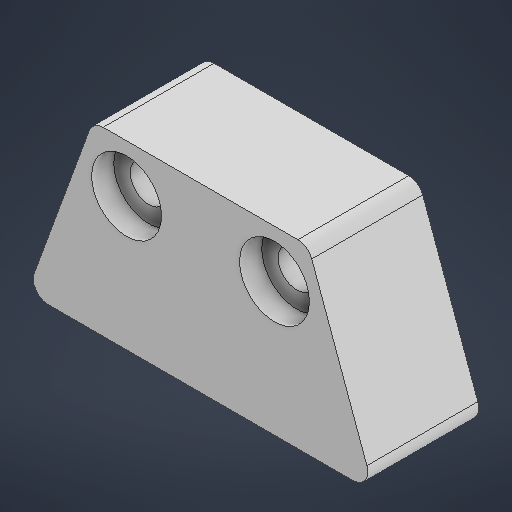
# Autodesk Inventor part: EngineMount
Saved by Autodesk Inventor 2025.3 (Build 293356030, 356C)
## iProperties
Created: 2025-10-14
Part Number: EngineMount
Material: Generic
Document SubType Name: Modeling
Designer: yo
Density: 1 g/cm^3
Appearance: Default
Author: yo
Autodesk Inventor part; units mm, degrees
ref_plane "YZ Plane" through (0, 0, 0) normal (1, 0, 0) x (0, 1, 0)
ref_plane "XZ Plane" through (0, 0, 0) normal (0, 1, 0) x (-1, 0, 0)
ref_plane "XY Plane" through (0, 0, 0) normal (0, 0, 1) x (1, 0, 0)
sketch "Sketch1" plane through (0, 0, 0) normal (0, 0, 1) x (1, 0, 0)
  line L0 (-41.2246, 0) -> (41.2246, 0)
  line L1 (-26.3201, 48.95) -> (26.3201, 48.95)
  circle A0 centre (-20, 36) radius 9.45
  line L2 (0, 48.95) -> (0, 0) construction
  circle A1 centre (-20, 36) radius 5
  circle A2 centre (20, 36) radius 9.45
  circle A3 centre (20, 36) radius 5
  arc A4 (-44.9834, 5.3681) -> (-41.2246, 0) centre (-41.2246, 4) ccw
  arc A5 (-26.3201, 48.95) -> (-30.0788, 46.3181) centre (-26.3201, 44.95) ccw
  line L3 (-44.9834, 5.3681) -> (-30.0788, 46.3181)
  arc A6 (41.2246, 0) -> (44.9834, 5.3681) centre (41.2246, 4) ccw
  arc A7 (30.0788, 46.3181) -> (26.3201, 48.95) centre (26.3201, 44.95) ccw
  line L4 (44.9834, 5.3681) -> (30.0788, 46.3181)
  dimension "d1" = 18.9
  dimension "d3" = 3.5
  dimension "d4" = 36
  dimension "d7" = 10
  dimension "d8" = 40
  dimension "d10" = 4
  dimension "d11" = 13
  dimension "d12" = 70
  constraints: 10 end point, 8 centre point, 8 point on circle, 6 symmetric about line, 4 coincident, 4 tangent, 2 horizontal, 2 midpoint, 1 equal radius, 1 vertical, 4 other
  measures "d1" diameter of A0
  measures "d3" distance edge to line of A0 L1
  measures "d4" distance from line of L0 A0.centre
  measures "d7" diameter of A1
  measures "d8" distance of A2.centre A0.centre
  measures "d10" radius of A4
  measures "d11" distance from line of A0.centre L3
  measures "d12" angle of L0 L3
extrude "Extrusion1" add sketch "Sketch1" along normal mid plane 30 contours A4 L3 A5 L1 A7 L4 A6 L0
extrude "Extrusion2" add sketch "Sketch1" along normal mid plane 18 contours A0 | A2
body "Solid1"
